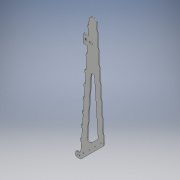
# Autodesk Inventor part: nowy_bok
Saved by Autodesk Inventor 2017 (Build 210142000, 142)
## iProperties
Created: 2019-10-28
Part Number: nowy_bok
Material: Ogólny
Document SubType Name: Modeling
Designer: patry
Density: 1 g/cm^3
Appearance: Domyślna
Author: patry
Autodesk Inventor part; units mm, degrees
ref_plane "YZ Plane" through (0, 0, 0) normal (1, 0, 0) x (0, 1, 0)
ref_plane "XZ Plane" through (0, 0, 0) normal (0, 1, 0) x (-1, 0, 0)
ref_plane "XY Plane" through (0, 0, 0) normal (0, 0, 1) x (1, 0, 0)
sketch "Szkic1" plane through (0, 0, 0) normal (0, 1, 0) x (-1, 0, 0)
  line L0 (-19, 622) -> (11, 622) construction
  line L1 (11, 622) -> (147, 486) construction
  line L2 (147, 486) -> (176.8016, 486) construction
  line L3 (176.8016, 486) -> (176.8016, 461) construction
  line L4 (-19, 622) -> (-19, 609.2855) construction
  line L5 (-19, 609.2855) -> (176.8016, 413.4839) construction
  line L6 (176.8016, 413.4839) -> (176.8016, 461) construction
  line L7 (176.8016, 486) -> (176.8016, 1189) construction
  line L8 (146.8016, 1189) -> (146.8016, 533) construction
  line L9 (246.8016, 495.9837) -> (246.8016, 1189) construction
  line L10 (-47, 922) -> (309, 922) construction
  line L11 (-42, 1147) -> (293, 1147) construction
  line L12 (12.455, 587.5586) -> (52.6586, 1162.4969)
  line L13 (67.6221, 1176.4505) -> (79.6466, 1176.4505)
  line L14 (147, 486) -> (147, 443.2855) construction
  line L15 (147, 486) -> (142.6159, 490.3841) construction
  line L16 (142.6159, 490.3841) -> (121.2587, 469.0268) construction
  line L17 (18.2642, 572.0213) -> (139.5006, 450.7849)
  line L18 (-99.7145, 690) -> (195.2855, 395) construction
  line L19 (172.3089, 417.9767) -> (172.3089, 447.856) construction
  line L20 (176.8016, 486) -> (315.5485, 347.2531) construction
  line L21 (141.5331, 491.4664) -> (138.3972, 536.3123)
  line L22 (162.3089, 477.5127) -> (156.4966, 477.5127)
  line L23 (162.3089, 447.856) -> (146.5717, 447.856)
  arc A0 (12.455, 587.5586) -> (18.2642, 572.0213) centre (32.4063, 586.1635) ccw
  line L24 (142.4296, 447.856) -> (172.3089, 417.9767) construction
  line L25 (172.3089, 457.856) -> (172.3089, 467.5127)
  arc A1 (141.5331, 491.4664) -> (156.4966, 477.5127) centre (156.4966, 492.5127) ccw
  arc A2 (172.3089, 467.5127) -> (162.3089, 477.5127) centre (162.3089, 467.5127) ccw
  arc A3 (162.3089, 447.856) -> (172.3089, 457.856) centre (162.3089, 457.856) ccw
  arc A4 (139.5006, 450.7849) -> (146.5717, 447.856) centre (146.5717, 457.856) ccw
  arc A5 (94.6101, 1162.4969) -> (79.6466, 1176.4505) centre (79.6466, 1161.4505) ccw
  arc A6 (67.6221, 1176.4505) -> (52.6586, 1162.4969) centre (67.6221, 1161.4505) ccw
  line L26 (141.5331, 491.4664) -> (144.7446, 445.541) construction
  line L27 (141.5331, 491.4664) -> (141.5331, 448.7524) construction
  line L28 (-28.6025, 640.2452) -> (163.5033, 448.1395) construction
  line L29 (47.7855, 542.5) -> (47.7855, 585.2145) construction
  line L30 (-4, 664.8499) -> (-4, 551.9978) construction
  line L31 (11, 622) -> (11, 579.2855) construction
  line L32 (11, 579.2855) -> (15.3841, 574.9015) construction
  line L33 (15.3841, 574.9015) -> (36.7413, 596.2587) construction
  line L34 (161.8016, 495.9837) -> (161.8016, 402) construction
  line L35 (104.2165, 1025.1187) -> (100.7287, 1074.9969) construction
  line L36 (100.7287, 1074.9969) -> (125.6678, 1076.7408)
  line L37 (125.6678, 1076.7408) -> (129.1556, 1026.8626)
  line L38 (129.1556, 1026.8626) -> (104.2165, 1025.1187)
  line L39 (100.7287, 1074.9969) -> (97.9384, 1114.8994)
  line L40 (104.2165, 1025.1187) -> (100.7287, 1074.9969) construction
  line L41 (73.1142, 1047.0024) -> (72.9747, 1048.9975)
  line L42 (74.8303, 1051.1322) -> (91.7889, 1052.318)
  line L43 (93.9236, 1050.4624) -> (94.0631, 1048.4673)
  line L44 (92.2075, 1046.3326) -> (75.2489, 1045.1468)
  line L45 (93.9933, 1049.4649) -> (102.4726, 1050.0578) construction
  line L46 (102.4726, 1050.0578) -> (114.4434, 1050.8949) construction
  arc A7 (74.8303, 1051.1322) -> (72.9747, 1048.9975) centre (74.9699, 1049.137) ccw
  arc A8 (73.1142, 1047.0024) -> (75.2489, 1045.1468) centre (75.1094, 1047.1419) ccw
  arc A9 (93.9236, 1050.4624) -> (91.7889, 1052.318) centre (91.9284, 1050.3229) ccw
  arc A10 (92.2075, 1046.3326) -> (94.0631, 1048.4673) centre (92.068, 1048.3278) ccw
  line L47 (116.505, 1021.4131) -> (111.1905, 1097.4131) construction
  line L48 (114.9666, 1043.4131) -> (113.9202, 1058.3766) construction
  line L49 (118.2139, 1047.1488) -> (117.6558, 1055.1293)
  line L50 (110.6729, 1054.641) -> (111.2309, 1046.6605)
  arc A11 (111.2309, 1046.6605) -> (118.2139, 1047.1488) centre (114.7224, 1046.9046) ccw
  arc A12 (117.6558, 1055.1293) -> (110.6729, 1054.641) centre (114.1644, 1054.8851) ccw
  line L51 (47.9957, 591.7873) -> (80.3202, 559.4628)
  line L52 (105.8902, 571.1158) -> (83.3114, 894.0086)
  line L53 (75.3309, 901.4505) -> (71.9379, 901.4505)
  line L54 (63.9574, 894.0086) -> (43.6388, 603.4402)
  arc A13 (43.6388, 603.4402) -> (47.9957, 591.7873) centre (58.6023, 602.3939) ccw
  arc A14 (80.3202, 559.4628) -> (105.8902, 571.1158) centre (90.9268, 570.0694) ccw
  arc A15 (83.3114, 894.0086) -> (75.3309, 901.4505) centre (75.3309, 893.4505) ccw
  arc A16 (71.9379, 901.4505) -> (63.9574, 894.0086) centre (71.9379, 893.4505) ccw
  line L55 (97.9384, 1114.8994) -> (96.8921, 1129.8629) construction
  line L56 (96.8921, 1129.8629) -> (101.8799, 1130.2117)
  line L57 (101.8799, 1130.2117) -> (102.9263, 1115.2482)
  line L58 (102.9263, 1115.2482) -> (97.9384, 1114.8994)
  line L59 (97.9384, 1114.8994) -> (112.9384, 1114.8994) construction
  line L60 (97.9384, 1114.8994) -> (96.8921, 1129.8629) construction
  line L61 (96.8921, 1129.8629) -> (94.6101, 1162.4969)
  line L62 (107.0068, 985.2161) -> (111.9946, 985.5649)
  line L63 (111.9946, 985.5649) -> (113.041, 970.6014)
  line L64 (113.041, 970.6014) -> (108.0531, 970.2527)
  line L65 (107.0068, 985.2161) -> (104.2165, 1025.1187)
  line L66 (108.0531, 970.2527) -> (107.0068, 985.2161) construction
  line L67 (138.3972, 536.3123) -> (137.3509, 551.2758)
  line L68 (137.3509, 551.2758) -> (143.3362, 551.6943)
  line L69 (143.3362, 551.6943) -> (144.3826, 536.7308)
  line L70 (144.3826, 536.7308) -> (138.3972, 536.3123)
  line L71 (138.3972, 536.3123) -> (153.3972, 536.3123) construction
  line L72 (131.9463, 1052.1188) -> (62.9796, 1047.2962) construction
  line L73 (137.3509, 551.2758) -> (108.0531, 970.2527)
  line L74 (138.3972, 536.3123) -> (137.3509, 551.2758) construction
  line L75 (138.4533, 621.5238) -> (139.4996, 606.5603)
  line L76 (139.4996, 606.5603) -> (133.5142, 606.1418)
  line L77 (132.4679, 621.1052) -> (138.4533, 621.5238)
  line L78 (133.5142, 606.1418) -> (132.4679, 621.1052)
  line L79 (133.5703, 691.3533) -> (134.6167, 676.3898)
  line L80 (134.6167, 676.3898) -> (128.6313, 675.9713)
  line L81 (127.5849, 690.9347) -> (133.5703, 691.3533)
  line L82 (128.6313, 675.9713) -> (127.5849, 690.9347)
  line L83 (128.6874, 761.1827) -> (129.7337, 746.2193)
  line L84 (129.7337, 746.2193) -> (123.7483, 745.8007)
  line L85 (122.702, 760.7642) -> (128.6874, 761.1827)
  line L86 (123.7483, 745.8007) -> (122.702, 760.7642)
  line L87 (123.8044, 831.0122) -> (124.8508, 816.0488)
  line L88 (124.8508, 816.0488) -> (118.8654, 815.6302)
  line L89 (117.819, 830.5937) -> (123.8044, 831.0122)
  line L90 (118.8654, 815.6302) -> (117.819, 830.5937)
  line L91 (118.9215, 900.8417) -> (119.9678, 885.8783)
  line L92 (119.9678, 885.8783) -> (113.9824, 885.4597)
  line L93 (112.9361, 900.4232) -> (118.9215, 900.8417)
  line L94 (113.9824, 885.4597) -> (112.9361, 900.4232)
  point P0 (0, 0)
  point P1 (11.8192, 578.4663)
  point P2 (53.6344, 1176.4505)
  point P3 (93.6344, 1176.4505)
  point P4 (172.3089, 477.5127)
  point P5 (142.5089, 477.5127)
  point P6 (47.7855, 563.8572)
  point P7 (27.4914, 584.1513)
  point P8 (148.7868, 462.856)
  point P9 (158.9877, 462.856)
  point P10 (93.2396, 518.4032)
  point P11 (60.3655, 551.2773)
  point P12 (126.1136, 485.5291)
  point P13 (72.8352, 1050.9927)
  point P14 (93.7841, 1052.4575)
  point P15 (118.4866, 1051.1776)
  dimension "d0" = 30
  dimension "d1" = 100
  dimension "d2" = 225
  dimension "d3" = 300
  dimension "d4" = 40
  dimension "d5" = 6.2
  dimension "d14" = 94
  dimension "d16" = 94
  dimension "d18" = 29.8
  dimension "d22" = 700.6445
  dimension "d23" = 20
  dimension "d24" = 15
  dimension "d25" = 10
  dimension "d26" = 10
  dimension "d28" = 15.7372
  dimension "d29" = 15
  dimension "d30" = 42.714
  dimension "d31" = 42.7145
  dimension "d32" = 21.3572
  dimension "d33" = 30
  dimension "d34" = 15
  dimension "d35" = 6.2
  dimension "d39" = 15.0364
  dimension "d40" = 15
  dimension "d43" = 23.5221
  dimension "d45" = 13.3212
  dimension "d46" = 15
  dimension "d47" = 131.4963
  dimension "d48" = 65.7481
  dimension "d49" = 32.8741
  dimension "d50" = 32.8741
  dimension "d51" = 50
  dimension "d52" = 25
  dimension "d53" = 87.5
  dimension "d56" = 21
  dimension "d57" = 8.5
  dimension "d58" = 12
  dimension "d60" = 2
  dimension "d62" = 6
  dimension "d63" = 15
  dimension "d64" = 7
  dimension "d65" = 25
  dimension "d66" = 275
  dimension "d67" = 30
  dimension "d68" = 30
  dimension "d69" = 35
  dimension "d70" = 15
  dimension "d71" = 8
  dimension "d72" = 15
  dimension "d73" = 94
  dimension "d74" = 5
  dimension "d75" = 40
  dimension "d78" = 145
  dimension "d83" = 15
  dimension "d84" = 94
  dimension "d85" = 6
  dimension "d86" = 3
  dimension "d87" = 16.014
  dimension "d88" = 25
  dimension "d99" = 70
  dimension "d113" = 420
  constraints: 190 end point, 51 tangent, 38 point on line, 36 point on circle, 25 parallel, 18 collinear, 17 centre point, 11 vertical, 9 perpendicular, 8 horizontal, 7 equal radius, 5 midpoint, 2 equal length, 59 other
  measures "d0" distance between parallel lines of L7 L8
  measures "d1" distance between parallel lines of L8 L9
  measures "d2" distance between parallel lines of L11 L10
  measures "d3" distance between parallel lines of L0 L10
  measures "d4" distance of point (53.634, 1176.451) point (93.634, 1176.451)
  measures "d5" distance of L1.end L15.end
  measures "d14" angle of L13 L12
  measures "d16" angle of L21 L13
  measures "d18" distance of point (172.309, 477.513) point (142.509, 477.513)
  measures "d22" distance of point (142.509, 477.513) point (93.634, 1176.451)
  measures "d23" radius of A0
  measures "d24" radius of A1
  measures "d25" radius of A2
  measures "d26" radius of A3
  measures "d28" distance of L23.start L23.end
  measures "d29" radius of A5
  measures "d30" distance of L21.start L27.end
  measures "d31" distance of L29.start L29.end
  measures "d32" distance of point (47.786, 563.857) L29.end
  measures "d33" distance of L0.end L0.start
  measures "d35" distance of L31.end L32.end
  measures "d39" horizontal distance of point (27.491, 584.151) L12.start
  measures "d40" distance between parallel lines of L3 L34
  measures "d43" distance from line of L25 point (148.787, 462.856)
  measures "d45" distance from line of L25 point (158.988, 462.856)
  measures "d46" distance from line of L23 point (158.988, 462.856)
  measures "d47" horizontal distance of point (158.988, 462.856) point (27.491, 584.151)
  measures "d48" horizontal distance of point (27.491, 584.151) point (93.24, 518.403)
  measures "d49" horizontal distance of point (60.365, 551.277) point (93.24, 518.403)
  measures "d50" horizontal distance of point (93.24, 518.403) point (126.114, 485.529)
  measures "d51" distance of L35.start L35.end
  measures "d52" distance of L35.end L36.end
  measures "d53" vertical distance of L61.end L35.end
  measures "d56" distance of point (72.835, 1050.993) point (93.784, 1052.458)
  measures "d57" distance of L45.start L45.end
  measures "d58" distance of L46.end L45.end
  measures "d60" radius of A7
  measures "d62" distance between parallel lines of L42 L44
  measures "d63" distance of L48.start L48.end
  measures "d64" diameter of A12
  measures "d65" distance from line of L35.end L45
  measures "d66" distance between parallel lines of L13 L53
  measures "d67" distance between parallel lines of L12 L54
  measures "d68" distance between parallel lines of L21 L52
  measures "d69" distance between parallel lines of L5 L51
  measures "d70" radius of A13
  measures "d71" radius of A15
  measures "d72" distance of L39.end L55.end
  measures "d73" angle of L59 L55
  measures "d74" distance of L55.end L56.end
  measures "d75" distance between parallel lines of L36 L58
  measures "d78" distance of L55.end L62.start
  measures "d83" distance of L21.end L67.end
  measures "d84" angle of L71 L67
  measures "d85" distance of L67.end L68.end
  measures "d86" distance between parallel lines of L42 L72
  measures "d87" horizontal distance of L45.end point (118.487, 1051.178)
  measures "d88" distance from line of L36 point (118.487, 1051.178)
  measures "d99" distance of L68.end L75.start
  measures "d113" distance between parallel lines of L68 L64
extrude "Wyciągnięcie proste1" add sketch "Szkic1" along normal blind 5
hole "Otwór1" at (-27.4914, 0, 584.1513) at (-148.7868, 0, 462.856) at (-158.9877, 0, 462.856) at (-93.2396, 0, 518.4032) at (-60.3655, 0, 551.2773) at (-126.1136, 0, 485.5291) direction (0, 1, 0) diameter 4.5 depth 8 tip angle 118 clearance for "Śruba ze łbem płaskim obrobiona" size "M4" standard "ANSI Profil metryczny M"
equation "\"d16\" = d14"
